Autodesk Inventor part; units mm, degrees
(part 2 of 2)
  spline S102 degree 2 poles (49.405, 85.2226) (49.2693, 85.2647) (48.9493, 85.4036) (48.8491, 85.4553) knots 0 0 0 1 2 2 2
  line L215 (48.8491, 85.4553) -> (48.8491, 86.4054)
  line L216 (48.8491, 86.4054) -> (48.9493, 86.4054)
  spline S103 degree 2 poles (48.9493, 86.4054) (49.0237, 86.3408) (49.2434, 86.1598) (49.3824, 86.0758) knots 0 0 0 1 2 2 2
  spline S104 degree 2 poles (49.3824, 86.0758) (49.5213, 85.9885) (49.8542, 85.869) (50.0384, 85.869) knots 0 0 0 1 2 2 2
  spline S105 degree 2 poles (50.0384, 85.869) (50.2549, 85.869) (50.6136, 86.0047) (50.7784, 86.176) knots 0 0 0 1 2 2 2
  spline S106 degree 2 poles (50.7784, 86.176) (50.9271, 86.3279) (51.1177, 86.8481) (51.1177, 87.2004) knots 0 0 0 1 2 2 2
  spline S107 degree 2 poles (51.1177, 87.2004) (51.1177, 87.572) (50.9206, 88.0794) (50.759, 88.2345) knots 0 0 0 1 2 2 2
  spline S108 degree 2 poles (50.759, 88.2345) (50.6039, 88.3864) (50.2226, 88.5189) (50.0319, 88.5189) knots 0 0 0 1 2 2 2
  spline S109 degree 2 poles (50.0319, 88.5189) (49.8348, 88.5189) (49.4761, 88.3864) (49.3533, 88.3056) knots 0 0 0 1 2 2 2
  spline S110 degree 2 poles (49.3533, 88.3056) (49.2176, 88.2248) (49.014, 88.0535) (48.9396, 87.9857) knots 0 0 0 1 2 2 2
  line L217 (48.9396, 87.9857) -> (48.8491, 87.9857)
  line L218 (48.8491, 87.9857) -> (48.8491, 88.9228)
  spline S111 degree 2 poles (48.8491, 88.9228) (48.959, 88.9745) (49.2466, 89.1038) (49.4018, 89.149) knots 0 0 0 1 2 2 2
  spline S112 degree 2 poles (49.4018, 89.149) (49.5892, 89.2072) (49.9156, 89.2654) (50.2, 89.2654) knots 0 0 0 1 2 2 2
  line L219 (46.6032, 87.7982) -> (48.3773, 87.7982)
  line L220 (48.3773, 87.7982) -> (48.3773, 87.055)
  line L221 (48.3773, 87.055) -> (46.6032, 87.055)
  line L222 (46.6032, 87.055) -> (46.6032, 87.7982)
  spline S113 degree 2 poles (42.3342, 87.1972) (42.3342, 87.7562) (42.8222, 88.6352) (43.1938, 88.8711) knots 0 0 0 1 2 2 2
  spline S114 degree 2 poles (43.1938, 88.8711) (43.5041, 89.0715) (44.2344, 89.1878) (44.6448, 89.1878) knots 0 0 0 1 2 2 2
  line L223 (44.6448, 89.1878) -> (45.8922, 89.1878)
  line L224 (45.8922, 89.1878) -> (45.8922, 85.2)
  line L225 (45.8922, 85.2) -> (44.6578, 85.2)
  spline S115 degree 2 poles (44.6578, 85.2) (44.2376, 85.2) (43.5041, 85.3067) (43.1809, 85.5135) knots 0 0 0 1 2 2 2
  spline S116 degree 2 poles (43.1809, 85.5135) (42.7899, 85.7656) (42.3342, 86.6187) (42.3342, 87.1972) knots 0 0 0 1 2 2 2
  spline S117 degree 2 poles (43.3619, 87.1907) (43.3619, 86.7964) (43.6333, 86.2341) (43.9113, 86.0758) knots 0 0 0 1 2 2 2
  spline S118 degree 2 poles (43.9113, 86.0758) (44.1148, 85.9659) (44.5608, 85.9433) (44.871, 85.9433) knots 0 0 0 1 2 2 2
  line L226 (44.871, 85.9433) -> (44.8904, 85.9433)
  line L227 (44.8904, 85.9433) -> (44.8904, 88.4413)
  line L228 (44.8904, 88.4413) -> (44.871, 88.4413)
  spline S119 degree 2 poles (44.871, 88.4413) (44.535, 88.4413) (44.0728, 88.4187) (43.8628, 88.2862) knots 0 0 0 1 2 2 2
  spline S120 degree 2 poles (43.8628, 88.2862) (43.6172, 88.1311) (43.3619, 87.5849) (43.3619, 87.1907) knots 0 0 0 1 2 2 2
  spline S121 degree 2 poles (40.0204, 89.2654) (40.9188, 89.2654) (41.9723, 88.1796) (41.9723, 87.1972) knots 0 0 0 1 2 2 2
  spline S122 degree 2 poles (41.9723, 87.1972) (41.9723, 86.2503) (40.9156, 85.1225) (40.0172, 85.1225) knots 0 0 0 1 2 2 2
  spline S123 degree 2 poles (40.0172, 85.1225) (39.7813, 85.1225) (39.3999, 85.1774) (39.2254, 85.2226) knots 0 0 0 1 2 2 2
  spline S124 degree 2 poles (39.2254, 85.2226) (39.0897, 85.2647) (38.7698, 85.4036) (38.6696, 85.4553) knots 0 0 0 1 2 2 2
  line L229 (38.6696, 85.4553) -> (38.6696, 86.4054)
  line L230 (38.6696, 86.4054) -> (38.7698, 86.4054)
  spline S125 degree 2 poles (38.7698, 86.4054) (38.8441, 86.3408) (39.0639, 86.1598) (39.2028, 86.0758) knots 0 0 0 1 2 2 2
  spline S126 degree 2 poles (39.2028, 86.0758) (39.3418, 85.9885) (39.6746, 85.869) (39.8588, 85.869) knots 0 0 0 1 2 2 2
  spline S127 degree 2 poles (39.8588, 85.869) (40.0753, 85.869) (40.4341, 86.0047) (40.5989, 86.176) knots 0 0 0 1 2 2 2
  spline S128 degree 2 poles (40.5989, 86.176) (40.7475, 86.3279) (40.9382, 86.8481) (40.9382, 87.2004) knots 0 0 0 1 2 2 2
  spline S129 degree 2 poles (40.9382, 87.2004) (40.9382, 87.572) (40.7411, 88.0794) (40.5795, 88.2345) knots 0 0 0 1 2 2 2
  spline S130 degree 2 poles (40.5795, 88.2345) (40.4244, 88.3864) (40.043, 88.5189) (39.8524, 88.5189) knots 0 0 0 1 2 2 2
  spline S131 degree 2 poles (39.8524, 88.5189) (39.6552, 88.5189) (39.2965, 88.3864) (39.1737, 88.3056) knots 0 0 0 1 2 2 2
  spline S132 degree 2 poles (39.1737, 88.3056) (39.038, 88.2248) (38.8344, 88.0535) (38.7601, 87.9857) knots 0 0 0 1 2 2 2
  line L231 (38.7601, 87.9857) -> (38.6696, 87.9857)
  line L232 (38.6696, 87.9857) -> (38.6696, 88.9228)
  spline S133 degree 2 poles (38.6696, 88.9228) (38.7795, 88.9745) (39.0671, 89.1038) (39.2222, 89.149) knots 0 0 0 1 2 2 2
  spline S134 degree 2 poles (39.2222, 89.149) (39.4096, 89.2072) (39.736, 89.2654) (40.0204, 89.2654) knots 0 0 0 1 2 2 2
  spline S135 degree 2 poles (35.2409, 89.2589) (35.6998, 89.2589) (36.3913, 89.0812) (36.6886, 88.9519) knots 0 0 0 1 2 2 2
  line L233 (36.6886, 88.9519) -> (36.6886, 88.0018)
  line L234 (36.6886, 88.0018) -> (36.5981, 88.0018)
  spline S136 degree 2 poles (36.5981, 88.0018) (36.2976, 88.2571) (35.5769, 88.5318) (35.2376, 88.5318) knots 0 0 0 1 2 2 2
  spline S137 degree 2 poles (35.2376, 88.5318) (35.1504, 88.5318) (34.8692, 88.493) (34.7852, 88.4542) knots 0 0 0 1 2 2 2
  spline S138 degree 2 poles (34.7852, 88.4542) (34.6818, 88.409) (34.5364, 88.2442) (34.5364, 88.1117) knots 0 0 0 1 2 2 2
  spline S139 degree 2 poles (34.5364, 88.1117) (34.5364, 87.9598) (34.7723, 87.7724) (34.9339, 87.7304) knots 0 0 0 1 2 2 2
  spline S140 degree 2 poles (34.9339, 87.7304) (35.1375, 87.6754) (35.5996, 87.5817) (35.8032, 87.5106) knots 0 0 0 1 2 2 2
  spline S141 degree 2 poles (35.8032, 87.5106) (36.2653, 87.349) (36.666, 86.7964) (36.666, 86.3828) knots 0 0 0 1 2 2 2
  spline S142 degree 2 poles (36.666, 86.3828) (36.666, 85.8237) (35.7191, 85.1289) (35.0082, 85.1289) knots 0 0 0 1 2 2 2
  spline S143 degree 2 poles (35.0082, 85.1289) (34.6527, 85.1289) (33.9482, 85.2743) (33.6703, 85.3971) knots 0 0 0 1 2 2 2
  line L235 (33.6703, 85.3971) -> (33.6703, 86.3085)
  line L236 (33.6703, 86.3085) -> (33.7576, 86.3085)
  spline S144 degree 2 poles (33.7576, 86.3085) (33.9805, 86.1178) (34.6204, 85.856) (34.9565, 85.856) knots 0 0 0 1 2 2 2
  spline S145 degree 2 poles (34.9565, 85.856) (35.089, 85.856) (35.2958, 85.8948) (35.4121, 85.9465) knots 0 0 0 1 2 2 2
  spline S146 degree 2 poles (35.4121, 85.9465) (35.5059, 85.9885) (35.6416, 86.1566) (35.6416, 86.26) knots 0 0 0 1 2 2 2
  spline S147 degree 2 poles (35.6416, 86.26) (35.6416, 86.4151) (35.4251, 86.5928) (35.1148, 86.6639) knots 0 0 0 1 2 2 2
  spline S148 degree 2 poles (35.1148, 86.6639) (34.9145, 86.7092) (34.5428, 86.7964) (34.3296, 86.8708) knots 0 0 0 1 2 2 2
  spline S149 degree 2 poles (34.3296, 86.8708) (33.9159, 87.0226) (33.512, 87.5268) (33.512, 87.9404) knots 0 0 0 1 2 2 2
  spline S150 degree 2 poles (33.512, 87.9404) (33.512, 88.535) (34.4459, 89.2589) (35.2409, 89.2589) knots 0 0 0 1 2 2 2
  spline S151 degree 2 poles (31.3856, 89.2718) (32.1902, 89.2718) (33.0563, 88.4963) (33.0563, 87.7465) knots 0 0 0 1 2 2 2
  line L237 (33.0563, 87.7465) -> (33.0563, 85.2)
  line L238 (33.0563, 85.2) -> (32.0545, 85.2)
  line L239 (32.0545, 85.2) -> (32.0545, 87.6884)
  spline S152 degree 2 poles (32.0545, 87.6884) (32.0545, 88.1052) (31.741, 88.5124) (31.3856, 88.5124) knots 0 0 0 1 2 2 2
  spline S153 degree 2 poles (31.3856, 88.5124) (31.0398, 88.5124) (30.7166, 88.1214) (30.7166, 87.6884) knots 0 0 0 1 2 2 2
  line L240 (30.7166, 87.6884) -> (30.7166, 85.2)
  line L241 (30.7166, 85.2) -> (29.7148, 85.2)
  line L242 (29.7148, 85.2) -> (29.7148, 87.7433)
  spline S154 degree 2 poles (29.7148, 87.7433) (29.7148, 88.4801) (30.5583, 89.2718) (31.3856, 89.2718) knots 0 0 0 1 2 2 2
  spline S155 degree 2 poles (25.8789, 86.4571) (25.8789, 86.735) (26.0566, 87.2392) (26.2215, 87.4072) knots 0 0 0 1 2 2 2
  spline S156 degree 2 poles (26.2215, 87.4072) (26.3216, 87.5139) (26.5672, 87.6884) (26.7127, 87.7498) knots 0 0 0 1 2 2 2
  spline S157 degree 2 poles (26.7127, 87.7498) (26.8613, 87.8112) (27.2071, 87.8823) (27.4204, 87.8823) knots 0 0 0 1 2 2 2
  line L243 (27.4204, 87.8823) -> (27.9439, 87.8823)
  line L244 (27.9439, 87.8823) -> (27.9439, 89.1878)
  line L245 (27.9439, 89.1878) -> (28.9457, 89.1878)
  line L246 (28.9457, 89.1878) -> (28.9457, 85.2)
  line L247 (28.9457, 85.2) -> (27.3978, 85.2)
  spline S158 degree 2 poles (27.3978, 85.2) (27.0552, 85.2) (26.5543, 85.3261) (26.3507, 85.4618) knots 0 0 0 1 2 2 2
  spline S159 degree 2 poles (26.3507, 85.4618) (26.1245, 85.6137) (25.8789, 86.1113) (25.8789, 86.4571) knots 0 0 0 1 2 2 2
  spline S160 degree 2 poles (26.9066, 86.483) (26.9066, 86.3117) (27.0681, 86.0693) (27.178, 86.0241) knots 0 0 0 1 2 2 2
  spline S161 degree 2 poles (27.178, 86.0241) (27.3202, 85.9627) (27.5787, 85.9433) (27.8017, 85.9433) knots 0 0 0 1 2 2 2
  line L248 (27.8017, 85.9433) -> (27.9439, 85.9433)
  line L249 (27.9439, 85.9433) -> (27.9439, 87.139)
  line L250 (27.9439, 87.139) -> (27.8728, 87.139)
  spline S162 degree 2 poles (27.8728, 87.139) (27.7338, 87.139) (27.4818, 87.1325) (27.3881, 87.1164) knots 0 0 0 1 2 2 2
  spline S163 degree 2 poles (27.3881, 87.1164) (27.3073, 87.1034) (27.1295, 87.0259) (27.0811, 86.9774) knots 0 0 0 1 2 2 2
  spline S164 degree 2 poles (27.0811, 86.9774) (26.9776, 86.8805) (26.9066, 86.6639) (26.9066, 86.483) knots 0 0 0 1 2 2 2
  spline S165 degree 2 poles (22.2757, 86.4571) (22.2757, 86.735) (22.4534, 87.2392) (22.6182, 87.4072) knots 0 0 0 1 2 2 2
  spline S166 degree 2 poles (22.6182, 87.4072) (22.7184, 87.5139) (22.964, 87.6884) (23.1094, 87.7498) knots 0 0 0 1 2 2 2
  spline S167 degree 2 poles (23.1094, 87.7498) (23.2581, 87.8112) (23.6039, 87.8823) (23.8171, 87.8823) knots 0 0 0 1 2 2 2
  line L251 (23.8171, 87.8823) -> (24.3407, 87.8823)
  line L252 (24.3407, 87.8823) -> (24.3407, 89.1878)
  line L253 (24.3407, 89.1878) -> (25.3425, 89.1878)
  line L254 (25.3425, 89.1878) -> (25.3425, 85.2)
  line L255 (25.3425, 85.2) -> (23.7945, 85.2)
  spline S168 degree 2 poles (23.7945, 85.2) (23.452, 85.2) (22.9511, 85.3261) (22.7475, 85.4618) knots 0 0 0 1 2 2 2
  spline S169 degree 2 poles (22.7475, 85.4618) (22.5213, 85.6137) (22.2757, 86.1113) (22.2757, 86.4571) knots 0 0 0 1 2 2 2
  spline S170 degree 2 poles (23.3033, 86.483) (23.3033, 86.3117) (23.4649, 86.0693) (23.5748, 86.0241) knots 0 0 0 1 2 2 2
  spline S171 degree 2 poles (23.5748, 86.0241) (23.717, 85.9627) (23.9755, 85.9433) (24.1985, 85.9433) knots 0 0 0 1 2 2 2
  line L256 (24.1985, 85.9433) -> (24.3407, 85.9433)
  line L257 (24.3407, 85.9433) -> (24.3407, 87.139)
  line L258 (24.3407, 87.139) -> (24.2696, 87.139)
  spline S172 degree 2 poles (24.2696, 87.139) (24.1306, 87.139) (23.8785, 87.1325) (23.7848, 87.1164) knots 0 0 0 1 2 2 2
  spline S173 degree 2 poles (23.7848, 87.1164) (23.704, 87.1034) (23.5263, 87.0259) (23.4778, 86.9774) knots 0 0 0 1 2 2 2
  spline S174 degree 2 poles (23.4778, 86.9774) (23.3744, 86.8805) (23.3033, 86.6639) (23.3033, 86.483) knots 0 0 0 1 2 2 2
  line L259 (19.0796, 89.1878) -> (21.7392, 89.1878)
  line L260 (21.7392, 89.1878) -> (21.7392, 85.2)
  line L261 (21.7392, 85.2) -> (20.7374, 85.2)
  line L262 (20.7374, 85.2) -> (20.7374, 88.4284)
  line L263 (20.7374, 88.4284) -> (19.0796, 88.4284)
  line L264 (19.0796, 88.4284) -> (19.0796, 89.1878)
  line L265 (15.2857, 85.2) -> (16.6624, 87.5235)
  line L266 (16.6624, 87.5235) -> (16.6624, 89.1878)
  line L267 (16.6624, 89.1878) -> (17.6642, 89.1878)
  line L268 (17.6642, 89.1878) -> (17.6642, 87.572)
  line L269 (17.6642, 87.572) -> (19.0635, 85.2)
  line L270 (19.0635, 85.2) -> (17.9227, 85.2)
  line L271 (17.9227, 85.2) -> (17.1439, 86.6219)
  line L272 (17.1439, 86.6219) -> (16.3909, 85.2)
  line L273 (16.3909, 85.2) -> (15.2857, 85.2)
  point P0 (70, 54.25)
  point P1 (134, 91.25)
  point P2 (134, 6.75)
  point P3 (132, 14)
  point P4 (134, 6.75)
  point P5 (141.5993, 15.6604)
  point P6 (11.2814, 15.6604)
  point P7 (124.6991, 15.6604)
  point P8 (70, 85.116)
  point P9 (3.9805, 86.4049)
  point P10 (6, 91.25)
  point P11 (134, 91.25)
  point P12 (70, 93)
  point P13 (70, 87.6939)
  dimension "d137" = 8
  dimension "d138" = 9
  constraints: 7 midpoint, 2 collinear, 2 horizontal alignment, 1 vertical alignment, 9 other
  measures "d137" distance from line of L12 point (132, 14)
  measures "d138" distance from line of L13 point (132, 14)
extrude "Extrusion20" cut sketch "Sketch13" against normal blind 1 bodies 2
chamfer "Chamfer1" distance 3 angle 45 8 edges at (75, 52, 5.25) (73.5355, 52, -42.2855) (0, 52, -43.75) (-73.5355, 52, -42.2855) (-75, 52, 5.25) (-73.5355, 52, 52.7855) (0, 52, 54.25) (73.5355, 52, 52.7855)
chamfer "Chamfer2" distance 2 angle 45 4 edges at (72, 49, 5.25) (0, 49, 51.25) (0, 49, -40.75) (-72, 49, 5.25)
chamfer "Chamfer3" distance 1 angle 45 4 edges at (71.5, 52, 47.5) (71.5, 52, -37) (-71.5, 52, 47.5) (-71.5, 52, -37)
sketch "Sketch14" plane through (75, 3, 49.25) normal (1, 0, 0) x (0, 0, -1)
  arc A0 (10.15, 3.35) -> (12.85, 3.35) centre (11.5, 3.35) ccw projected
  line L0 (10.15, 3.35) -> (10.15, 7) projected
  line L1 (12.85, 7) -> (12.85, 3.35) projected
  line L2 (14.2, 7) -> (14.2, 3.35)
  arc A1 (8.8, 3.35) -> (14.2, 3.35) centre (11.5, 3.35) ccw
  line L3 (8.8, 3.35) -> (8.8, 7)
  line L4 (8.8, 7) -> (14.2, 7)
  point P0 (49.25, -3)
  dimension "d150" = 1.35
  dimension "d151" = 1.35
  constraints: 6 end point, 2 point on circle, 1 centre point, 1 horizontal, 2 other
  measures "d150" radius of A0
  measures "d151" distance between parallel lines of L1 L2
sketch "Sketch15" plane through (-70, 52, 54.25) normal (0, 1, 0) x (1, 0, 0)
  arc A0 (-2, 89.25) -> (3.75, 95) centre (1.75, 91.25) ccw projected
  line L0 (-2, 8.75) -> (-2, 89.25) projected
  arc A1 (3.75, 3) -> (-2, 8.75) centre (1.75, 6.75) ccw projected
  line L1 (136.25, 3) -> (3.75, 3) projected
  arc A2 (142, 8.75) -> (136.25, 3) centre (138.25, 6.75) ccw projected
  line L2 (142, 89.25) -> (142, 8.75) projected
  arc A3 (136.25, 95) -> (142, 89.25) centre (138.25, 91.25) ccw projected
  line L3 (3.75, 95) -> (136.25, 95) projected
  line L4 (68.25, 73) -> (64.75, 76.5) projected
  line L5 (64.75, 76.5) -> (64.75, 56) projected
  line L6 (64.75, 56) -> (61.25, 56) projected
  line L7 (61.25, 56) -> (61.25, 81.5) projected
  line L8 (61.25, 81.5) -> (71.75, 81.5) projected
  line L9 (71.75, 81.5) -> (71.75, 63.25) projected
  line L10 (71.75, 63.25) -> (75.25, 59.75) projected
  line L11 (75.25, 59.75) -> (75.25, 81.5) projected
  line L12 (75.25, 81.5) -> (78.75, 81.5) projected
  line L13 (78.75, 81.5) -> (78.75, 56) projected
  line L14 (78.75, 56) -> (68.25, 56) projected
  line L15 (68.25, 56) -> (68.25, 73) projected
  line L16 (96.25, 76.5) -> (87.25, 76.5) projected
  line L17 (87.25, 76.5) -> (87.25, 56) projected
  line L18 (87.25, 56) -> (83, 56) projected
  line L19 (83, 56) -> (83, 81.5) projected
  line L20 (83, 81.5) -> (100.5, 81.5) projected
  line L21 (100.5, 81.5) -> (100.5, 56) projected
  line L22 (100.5, 56) -> (96.25, 56) projected
  line L23 (96.25, 56) -> (96.25, 76.5) projected
  line L24 (39.5, 63.5) -> (39.5, 81.5) projected
  line L25 (39.5, 81.5) -> (57, 81.5) projected
  line L26 (57, 81.5) -> (57, 56) projected
  line L27 (57, 56) -> (39.5, 56) projected
  line L28 (39.5, 56) -> (39.5, 59.75) projected
  line L29 (39.5, 59.75) -> (53.25, 59.75) projected
  line L30 (53.25, 59.75) -> (53.25, 76.5) projected
  line L31 (53.25, 76.5) -> (43.25, 76.5) projected
  line L32 (43.25, 76.5) -> (43.25, 67.25) projected
  line L33 (43.25, 67.25) -> (46, 67.25) projected
  line L34 (46, 67.25) -> (46, 63.5) projected
  line L35 (46, 63.5) -> (39.5, 63.5) projected
  line L36 (104.75, 65.7386) -> (104.75, 81.5) projected
  line L37 (104.75, 81.5) -> (122.25, 81.5) projected
  line L38 (122.25, 81.5) -> (122.25, 56) projected
  line L39 (122.25, 56) -> (104.75, 56) projected
  line L40 (104.75, 56) -> (104.75, 61.9886) projected
  line L41 (104.75, 61.9886) -> (108.5, 65.7386) projected
  line L42 (108.5, 65.7386) -> (104.75, 65.7386) projected
  line L43 (30, 68.25) -> (30, 81.5) projected
  line L44 (30, 81.5) -> (35.25, 81.5) projected
  line L45 (35.25, 81.5) -> (35.25, 56) projected
  line L46 (35.25, 56) -> (17.75, 56) projected
  line L47 (17.75, 56) -> (17.75, 81.5) projected
  line L48 (17.75, 81.5) -> (23, 81.5) projected
  line L49 (23, 81.5) -> (23, 68.25) projected
  line L50 (23, 68.25) -> (30, 68.25) projected
  line L51 (39.5, 48.5) -> (118, 48.5) projected
  line L52 (118, 48.5) -> (118, 32.4) projected
  line L53 (118, 32.4) -> (119, 32.4) projected
  line L54 (119, 32.4) -> (119, 20.1) projected
  line L55 (119, 20.1) -> (118, 20.1) projected
  line L56 (118, 20.1) -> (118, 4) projected
  line L57 (118, 4) -> (39.5, 4) projected
  line L58 (39.5, 4) -> (39.5, 20.1) projected
  line L59 (39.5, 20.1) -> (38.5, 20.1) projected
  line L60 (38.5, 20.1) -> (38.5, 32.4) projected
  line L61 (38.5, 32.4) -> (39.5, 32.4) projected
  line L62 (39.5, 32.4) -> (39.5, 48.5) projected
  line L63 (16.3909, 85.2) -> (15.2857, 85.2) projected
  line L64 (15.2857, 85.2) -> (16.6624, 87.5235) projected
  line L65 (16.6624, 87.5235) -> (16.6624, 89.1878) projected
  line L66 (16.6624, 89.1878) -> (17.6642, 89.1878) projected
  line L67 (17.6642, 89.1878) -> (17.6642, 87.572) projected
  line L68 (17.6642, 87.572) -> (19.0635, 85.2) projected
  line L69 (19.0635, 85.2) -> (17.9227, 85.2) projected
  line L70 (17.9227, 85.2) -> (17.1439, 86.6219) projected
  line L71 (17.1439, 86.6219) -> (16.3909, 85.2) projected
  line L72 (33.0563, 87.7465) -> (33.0563, 85.2) projected
  line L73 (33.0563, 85.2) -> (32.0545, 85.2) projected
  line L74 (32.0545, 85.2) -> (32.0545, 87.6884) projected
  line L75 (30.7166, 87.6884) -> (30.7166, 85.2) projected
  line L76 (30.7166, 85.2) -> (29.7148, 85.2) projected
  line L77 (29.7148, 85.2) -> (29.7148, 87.7433) projected
  line L78 (38.6696, 85.4553) -> (38.6696, 86.4054) projected
  line L79 (38.6696, 86.4054) -> (38.7698, 86.4054) projected
  line L80 (38.7601, 87.9857) -> (38.6696, 87.9857) projected
  line L81 (38.6696, 87.9857) -> (38.6696, 88.9228) projected
  line L82 (44.6448, 89.1878) -> (45.8922, 89.1878) projected
  line L83 (45.8922, 89.1878) -> (45.8922, 85.2) projected
  line L84 (45.8922, 85.2) -> (44.6578, 85.2) projected
  line L85 (48.8491, 85.4553) -> (48.8491, 86.4054) projected
  line L86 (48.8491, 86.4054) -> (48.9493, 86.4054) projected
  line L87 (48.9396, 87.9857) -> (48.8491, 87.9857) projected
  line L88 (48.8491, 87.9857) -> (48.8491, 88.9228) projected
  line L89 (54.8244, 89.1878) -> (56.0718, 89.1878) projected
  line L90 (56.0718, 89.1878) -> (56.0718, 85.2) projected
  line L91 (56.0718, 85.2) -> (54.8373, 85.2) projected
  line L92 (59.3163, 87.4912) -> (57.9752, 89.1878) projected
  line L93 (57.9752, 89.1878) -> (59.1935, 89.1878) projected
  line L94 (59.1935, 89.1878) -> (60.302, 87.7239) projected
  line L95 (60.302, 87.7239) -> (60.6639, 87.7239) projected
  line L96 (60.6639, 87.7239) -> (60.6639, 89.1878) projected
  line L97 (60.6639, 89.1878) -> (61.6592, 89.1878) projected
  line L98 (61.6592, 89.1878) -> (61.6592, 85.2) projected
  line L99 (61.6592, 85.2) -> (60.0564, 85.2) projected
  line L100 (65.8603, 85.2) -> (65.8603, 89.1878) projected
  line L101 (65.8603, 89.1878) -> (66.8556, 89.1878) projected
  line L102 (66.8556, 89.1878) -> (66.8556, 86.5444) projected
  line L103 (66.8556, 86.5444) -> (67.5795, 88.2507) projected
  line L104 (67.5795, 88.2507) -> (68.2646, 88.2507) projected
  line L105 (68.2646, 88.2507) -> (68.9885, 86.5444) projected
  line L106 (68.9885, 86.5444) -> (68.9885, 89.1878) projected
  line L107 (68.9885, 89.1878) -> (69.9321, 89.1878) projected
  line L108 (69.9321, 89.1878) -> (69.9321, 85.2) projected
  line L109 (69.9321, 85.2) -> (68.7785, 85.2) projected
  line L110 (68.7785, 85.2) -> (67.893, 87.1681) projected
  line L111 (67.893, 87.1681) -> (67.014, 85.2) projected
  line L112 (67.014, 85.2) -> (65.8603, 85.2) projected
  line L113 (71.5706, 87.4912) -> (70.2294, 89.1878) projected
  line L114 (70.2294, 89.1878) -> (71.4478, 89.1878) projected
  line L115 (71.4478, 89.1878) -> (72.5562, 87.7239) projected
  line L116 (72.5562, 87.7239) -> (72.9181, 87.7239) projected
  line L117 (72.9181, 87.7239) -> (72.9181, 89.1878) projected
  line L118 (72.9181, 89.1878) -> (73.9135, 89.1878) projected
  line L119 (73.9135, 89.1878) -> (73.9135, 85.2) projected
  line L120 (73.9135, 85.2) -> (72.3106, 85.2) projected
  line L121 (85.014, 88.9519) -> (85.014, 88.0018) projected
  line L122 (85.014, 88.0018) -> (84.9235, 88.0018) projected
  line L123 (81.9957, 85.3971) -> (81.9957, 86.3085) projected
  line L124 (81.9957, 86.3085) -> (82.083, 86.3085) projected
  line L125 (98.3509, 89.1878) -> (99.3527, 89.1878) projected
  line L126 (99.3527, 89.1878) -> (99.3527, 85.9594) projected
  line L127 (99.3527, 85.9594) -> (100.5322, 85.9594) projected
  line L128 (100.5322, 85.9594) -> (100.5322, 85.2) projected
  line L129 (100.5322, 85.2) -> (97.1713, 85.2) projected
  line L130 (97.1713, 85.2) -> (97.1713, 85.9594) projected
  line L131 (97.1713, 85.9594) -> (98.3509, 85.9594) projected
  line L132 (98.3509, 85.9594) -> (98.3509, 89.1878) projected
  line L133 (104.9078, 89.1878) -> (105.9096, 89.1878) projected
  line L134 (105.9096, 89.1878) -> (104.562, 85.2) projected
  line L135 (104.562, 85.2) -> (103.4697, 85.2) projected
  line L136 (103.4697, 85.2) -> (102.1221, 89.1878) projected
  line L137 (102.1221, 89.1878) -> (103.153, 89.1878) projected
  line L138 (103.153, 89.1878) -> (103.4019, 88.3735) projected
  line L139 (103.4019, 88.3735) -> (104.6557, 88.3735) projected
  line L140 (104.6557, 88.3735) -> (104.9078, 89.1878) projected
  line L141 (114.0694, 88.9519) -> (114.0694, 88.0018) projected
  line L142 (114.0694, 88.0018) -> (113.9789, 88.0018) projected
  line L143 (111.0511, 85.3971) -> (111.0511, 86.3085) projected
  line L144 (111.0511, 86.3085) -> (111.1383, 86.3085) projected
  line L145 (117.036, 89.1878) -> (118.0378, 89.1878) projected
  line L146 (118.0378, 89.1878) -> (116.6902, 85.2) projected
  line L147 (116.6902, 85.2) -> (115.5979, 85.2) projected
  line L148 (115.5979, 85.2) -> (114.2504, 89.1878) projected
  line L149 (114.2504, 89.1878) -> (115.2812, 89.1878) projected
  line L150 (115.2812, 89.1878) -> (115.5301, 88.3735) projected
  line L151 (115.5301, 88.3735) -> (116.7839, 88.3735) projected
  line L152 (116.7839, 88.3735) -> (117.036, 89.1878) projected
  line L153 (1.5417, 14) -> (1.5417, 19.9944) projected
  line L154 (1.5417, 19.9944) -> (2.9893, 19.9944) projected
  line L155 (2.9893, 19.9944) -> (5.3016, 15.8168) projected
  line L156 (5.3016, 15.8168) -> (5.3016, 19.9944) projected
  line L157 (5.3016, 19.9944) -> (6.6763, 19.9944) projected
  line L158 (6.6763, 19.9944) -> (6.6763, 14) projected
  line L159 (6.6763, 14) -> (4.8304, 14) projected
  line L160 (4.8304, 14) -> (2.9165, 17.4344) projected
  line L161 (2.9165, 17.4344) -> (2.9165, 14) projected
  line L162 (2.9165, 14) -> (1.5417, 14) projected
  line L163 (123.5814, 20.1207) -> (125.0873, 20.1207) projected
  line L164 (125.0873, 20.1207) -> (125.0873, 15.2679) projected
  line L165 (125.0873, 15.2679) -> (126.8604, 15.2679) projected
  line L166 (126.8604, 15.2679) -> (126.8604, 14.1263) projected
  line L167 (126.8604, 14.1263) -> (121.8084, 14.1263) projected
  line L168 (121.8084, 14.1263) -> (121.8084, 15.2679) projected
  line L169 (121.8084, 15.2679) -> (123.5814, 15.2679) projected
  line L170 (123.5814, 15.2679) -> (123.5814, 20.1207) projected
  line L171 (132.4176, 17.9542) -> (132.4176, 14.1263) projected
  line L172 (132.4176, 14.1263) -> (130.9117, 14.1263) projected
  line L173 (130.9117, 14.1263) -> (130.9117, 17.8667) projected
  line L174 (128.9006, 17.8667) -> (128.9006, 14.1263) projected
  line L175 (128.9006, 14.1263) -> (127.3947, 14.1263) projected
  line L176 (127.3947, 14.1263) -> (127.3947, 17.9493) projected
  line L177 (7.677, 18.95) -> (7.677, 19.9944) projected
  line L178 (7.677, 19.9944) -> (10.9025, 19.9944) projected
  line L179 (10.9025, 19.9944) -> (10.9025, 18.95) projected
  line L180 (10.9025, 18.95) -> (10.0427, 18.95) projected
  line L181 (10.0427, 18.95) -> (10.0427, 15.0444) projected
  line L182 (10.0427, 15.0444) -> (10.9025, 15.0444) projected
  line L183 (10.9025, 15.0444) -> (10.9025, 14) projected
  line L184 (10.9025, 14) -> (7.677, 14) projected
  line L185 (7.677, 14) -> (7.677, 15.0444) projected
  line L186 (7.677, 15.0444) -> (8.5368, 15.0444) projected
  line L187 (8.5368, 15.0444) -> (8.5368, 18.95) projected
  line L188 (8.5368, 18.95) -> (7.677, 18.95) projected
  line L189 (122.8238, 87.8823) -> (123.3473, 87.8823) projected
  line L190 (123.3473, 87.8823) -> (123.3473, 89.1878) projected
  line L191 (123.3473, 89.1878) -> (124.3491, 89.1878) projected
  line L192 (124.3491, 89.1878) -> (124.3491, 85.2) projected
  line L193 (124.3491, 85.2) -> (122.8012, 85.2) projected
  line L194 (118.0863, 88.4284) -> (118.0863, 89.1878) projected
  line L195 (118.0863, 89.1878) -> (120.7459, 89.1878) projected
  line L196 (120.7459, 89.1878) -> (120.7459, 85.2) projected
  line L197 (120.7459, 85.2) -> (119.7441, 85.2) projected
  line L198 (119.7441, 85.2) -> (119.7441, 88.4284) projected
  line L199 (119.7441, 88.4284) -> (118.0863, 88.4284) projected
  line L200 (106.3071, 85.2) -> (106.3071, 89.1878) projected
  line L201 (106.3071, 89.1878) -> (107.3024, 89.1878) projected
  line L202 (107.3024, 89.1878) -> (107.3024, 86.5444) projected
  line L203 (107.3024, 86.5444) -> (108.0263, 88.2507) projected
  line L204 (108.0263, 88.2507) -> (108.7114, 88.2507) projected
  line L205 (108.7114, 88.2507) -> (109.4353, 86.5444) projected
  line L206 (109.4353, 86.5444) -> (109.4353, 89.1878) projected
  line L207 (109.4353, 89.1878) -> (110.3789, 89.1878) projected
  line L208 (110.3789, 89.1878) -> (110.3789, 85.2) projected
  line L209 (110.3789, 85.2) -> (109.2252, 85.2) projected
  line L210 (109.2252, 85.2) -> (108.3398, 87.1681) projected
  line L211 (108.3398, 87.1681) -> (107.4608, 85.2) projected
  line L212 (107.4608, 85.2) -> (106.3071, 85.2) projected
  line L213 (91.9555, 88.3735) -> (92.2076, 89.1878) projected
  line L214 (92.2076, 89.1878) -> (94.2952, 89.1878) projected
  line L215 (94.2952, 89.1878) -> (95.4036, 87.7239) projected
  line L216 (95.4036, 87.7239) -> (95.7656, 87.7239) projected
  line L217 (95.7656, 87.7239) -> (95.7656, 89.1878) projected
  line L218 (95.7656, 89.1878) -> (96.7609, 89.1878) projected
  line L219 (96.7609, 89.1878) -> (96.7609, 85.2) projected
  line L220 (96.7609, 85.2) -> (95.158, 85.2) projected
  line L221 (94.418, 87.4912) -> (93.1697, 89.0704) projected
  line L222 (93.1697, 89.0704) -> (91.8618, 85.2) projected
  line L223 (91.8618, 85.2) -> (90.7695, 85.2) projected
  line L224 (90.7695, 85.2) -> (89.4219, 89.1878) projected
  line L225 (89.4219, 89.1878) -> (90.4528, 89.1878) projected
  line L226 (90.4528, 89.1878) -> (90.7017, 88.3735) projected
  line L227 (90.7017, 88.3735) -> (91.9555, 88.3735) projected
  line L228 (85.6086, 85.2) -> (85.6086, 89.1878) projected
  line L229 (85.6086, 89.1878) -> (86.5717, 89.1878) projected
  line L230 (86.5717, 89.1878) -> (88.1099, 86.4086) projected
  line L231 (88.1099, 86.4086) -> (88.1099, 89.1878) projected
  line L232 (88.1099, 89.1878) -> (89.0245, 89.1878) projected
  line L233 (89.0245, 89.1878) -> (89.0245, 85.2) projected
  line L234 (89.0245, 85.2) -> (87.7964, 85.2) projected
  line L235 (87.7964, 85.2) -> (86.5232, 87.4848) projected
  line L236 (86.5232, 87.4848) -> (86.5232, 85.2) projected
  line L237 (86.5232, 85.2) -> (85.6086, 85.2) projected
  line L238 (78.6542, 85.2) -> (78.6542, 85.9594) projected
  line L239 (78.6542, 85.9594) -> (80.3282, 85.9594) projected
  line L240 (80.3282, 85.9594) -> (80.3282, 86.7124) projected
  line L241 (80.3282, 86.7124) -> (78.7867, 86.7124) projected
  line L242 (78.7867, 86.7124) -> (78.7867, 87.4718) projected
  line L243 (78.7867, 87.4718) -> (80.3282, 87.4718) projected
  line L244 (80.3282, 87.4718) -> (80.3282, 89.1878) projected
  line L245 (80.3282, 89.1878) -> (81.3235, 89.1878) projected
  line L246 (81.3235, 89.1878) -> (81.3235, 85.2) projected
  line L247 (81.3235, 85.2) -> (78.6542, 85.2) projected
  line L248 (62.3379, 89.1878) -> (65.033, 89.1878) projected
  line L249 (65.033, 89.1878) -> (65.033, 85.2) projected
  line L250 (65.033, 85.2) -> (62.3379, 85.2) projected
  line L251 (62.3379, 85.2) -> (62.3379, 85.9594) projected
  line L252 (62.3379, 85.9594) -> (64.0377, 85.9594) projected
  line L253 (64.0377, 85.9594) -> (64.0377, 86.6607) projected
  line L254 (64.0377, 86.6607) -> (62.4704, 86.6607) projected
  line L255 (62.4704, 86.6607) -> (62.4704, 87.4201) projected
  line L256 (62.4704, 87.4201) -> (64.0377, 87.4201) projected
  line L257 (64.0377, 87.4201) -> (64.0377, 88.4284) projected
  line L258 (64.0377, 88.4284) -> (62.3379, 88.4284) projected
  line L259 (62.3379, 88.4284) -> (62.3379, 89.1878) projected
  line L260 (46.6032, 87.055) -> (46.6032, 87.7982) projected
  line L261 (46.6032, 87.7982) -> (48.3773, 87.7982) projected
  line L262 (48.3773, 87.7982) -> (48.3773, 87.055) projected
  line L263 (48.3773, 87.055) -> (46.6032, 87.055) projected
  line L264 (36.6886, 88.9519) -> (36.6886, 88.0018) projected
  line L265 (36.6886, 88.0018) -> (36.5981, 88.0018) projected
  line L266 (33.6703, 85.3971) -> (33.6703, 86.3085) projected
  line L267 (33.6703, 86.3085) -> (33.7576, 86.3085) projected
  line L268 (27.4204, 87.8823) -> (27.9439, 87.8823) projected
  line L269 (27.9439, 87.8823) -> (27.9439, 89.1878) projected
  line L270 (27.9439, 89.1878) -> (28.9457, 89.1878) projected
  line L271 (28.9457, 89.1878) -> (28.9457, 85.2) projected
  line L272 (28.9457, 85.2) -> (27.3978, 85.2) projected
  line L273 (23.8171, 87.8823) -> (24.3407, 87.8823) projected
  line L274 (24.3407, 87.8823) -> (24.3407, 89.1878) projected
  line L275 (24.3407, 89.1878) -> (25.3425, 89.1878) projected
  line L276 (25.3425, 89.1878) -> (25.3425, 85.2) projected
  line L277 (25.3425, 85.2) -> (23.7945, 85.2) projected
  line L278 (19.0796, 88.4284) -> (19.0796, 89.1878) projected
  line L279 (19.0796, 89.1878) -> (21.7392, 89.1878) projected
  line L280 (21.7392, 89.1878) -> (21.7392, 85.2) projected
  line L281 (21.7392, 85.2) -> (20.7374, 85.2) projected
  line L282 (20.7374, 85.2) -> (20.7374, 88.4284) projected
  line L283 (20.7374, 88.4284) -> (19.0796, 88.4284) projected
  point P0 (70, 54.25)
  constraints: 124 other
extrude "Extrusion22" add sketch "Sketch15" against normal up to surface (3 mm away) contours L51 L52 L53 L54 L55 L56 L57 L58 L59 L60 L61 L62 bodies 2
sketch "Sketch16" plane through (-70, 52, 54.25) normal (0, 1, 0) x (1, 0, 0)
  line L0 (110.8, 8) -> (29.2, 8)
  line L1 (29.2, 8) -> (29.2, 48.6)
  line L2 (29.2, 48.6) -> (110.8, 48.6)
  line L3 (110.8, 48.6) -> (110.8, 8)
  line L4 (136.25, 3) -> (3.75, 3) projected
  point P0 (70, 54.25)
  point P1 (70, 48.6)
  dimension "d156" = 40.6
  dimension "d157" = 81.6
  dimension "d158" = 5
  constraints: 8 end point, 2 parallel, 1 horizontal, 1 midpoint, 1 perpendicular, 1 vertical alignment
  measures "d156" distance of L2.end L0.start
  measures "d157" distance of L1.end L2.end
  measures "d158" distance between parallel lines of L4 L0
extrude "Extrusion23" cut sketch "Sketch16" against normal up to surface (3 mm away) bodies 2
equation "\"d4\" = dM3insert"
equation "\"d11\" = dM3boss"
equation "\"d69\" = dM3insert"
equation "\"d70\" = dM3boss"
equation "\"d81\" = dM3clearance"
equation "\"d82\" = M3headClearance"
equation "\"dM3insert\" = 4.2"
equation "\"d6\" = 4.1"
equation "\"d8\" = 4.1"
equation "\"d10\" = 4.1"
equation "\"d12\" = 4.1"
equation "\"dM3clearance\" = 3.4"
equation "\"dM3boss\" = 7.5"
equation "\"d14\" = 7.5"
equation "\"d73\" = 4.1"
equation "\"d74\" = 7.5"
equation "\"M3headClearance\" = 6.5"
